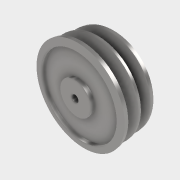
# Autodesk Inventor part: PWTR-0096
Saved by Autodesk Inventor 2021.1 (Build 251245000, 245)
## iProperties
CustomPartVersion: 1
Created: 2020-08-28
Part Number: PWTR-0096
Material: Stainless Steel
Document SubType Name: Modeling
Designer: alid
Density: 8 g/cm^3
Appearance: Semi-Polished
Description: Drive Unit Upper Pulley
Author: alid
Revision Number: A
Autodesk Inventor part; units mm, degrees
ref_plane "YZ Plane" through (0, 0, 0) normal (1, 0, 0) x (0, 1, 0)
ref_plane "XZ Plane" through (0, 0, 0) normal (0, 1, 0) x (-1, 0, 0)
sketch "Main Sketch" plane through (0, 0, 0) normal (1, 0, 0) x (0, 1, 0)
  line L0 (0, 28) -> (42, 28)
  line L1 (42, 28) -> (42, 12.8615)
  line L2 (42, 12.8615) -> (31, 9.4984)
  line L3 (31, 9.4984) -> (31, 6.5016)
  line L4 (31, 6.5016) -> (42, 3.1385)
  line L5 (42, 3.1385) -> (42, 0)
  line L6 (42, 0) -> (0, 0)
  line L7 (40, 12.25) -> (40, 3.75) construction
  line L8 (31, 8) -> (40, 8) construction
  line L9 (42, 12.8615) -> (42, 3.1385)
  line L10 (0, -5.6) -> (0, 33.6) projected
  line L11 (0, 0) -> (0, 28)
  line L12 (36, 0) -> (36, 3.5)
  line L13 (36, 3.5) -> (15, 3.5)
  line L14 (15, 3.5) -> (15, 0)
  line L15 (36, 28) -> (36, 24.5)
  line L16 (36, 24.5) -> (15, 24.5)
  line L17 (15, 24.5) -> (15, 28)
  dimension "d0" = 8.5
  dimension "d1" = 34
  dimension "d2" = 2
  dimension "d6" = 28
  dimension "d21" = 80
  dimension "d25" = 11
  dimension "d27" = 8
  dimension "d35" = 6
  dimension "d36" = 15
  dimension "d37" = 3.5
  constraints: 34 end point, 11 perpendicular, 6 point on line, 3 collinear, 2 equal length, 2 midpoint, 1 parallel
  measures "d0" distance of L7.start L7.end
  measures "d1" angle of L2 L4
  measures "d2" distance between parallel lines of L1 L7
  measures "d6" distance between parallel lines of L6 L0
  measures "d21" diameter of L7 L10
  measures "d25" distance between parallel lines of L3 L9
  measures "d27" distance between parallel lines of L6 L8
  measures "d35" distance between parallel lines of L5 L12
  measures "d36" distance between parallel lines of L10 L14
  measures "d37" distance of L13.end L14.end
ref_plane "Belt Plane" through (0, 31, 8) normal (0, 0, 1) x (1, 0, 0)
revolve "Body" add sketch "Main Sketch" angle 360 about axis through (0, 0, -10) along (0, 0, 1) contours L0 L17 L16 L15 L1 L2 L3 L4 L5 L6 L12 L13 L14 L10 | L9 L4 L3 L2
revolve "Groove" cut sketch "Main Sketch" angle 360 about axis through (0, 0, -10) along (0, 0, 1) contours L9 L4 L3 L2
fillet "Fillet External" [suppressed]
fillet "Fillet Internal" [suppressed]
pattern_linear "Groove Pattern" count 2 spacing 12 along (0, 0, 1) of "Groove"
sketch "Sketch2" plane through (0, 0, 0) normal (0, 0, -1) x (-1, 0, 0)
  circle A0 centre (0, 0) radius 42 projected
  constraints: 1 coincident
hole "Hole1" at (0, 0, 0) direction (0, 0, 1) diameter 6.6 end through all counterbore diameter 18 counterbore depth 23
equation "\"d0\" = da_Bw"
equation "\"d1\" = da_Alfa"
equation "\"d2\" = da_c"
equation "\"d21\" = da_Dw"
equation "\"d25\" = da_Hd"
equation "\"d27\" = da_Se"
equation "\"da_r1\" = 0"
equation "\"da_r2\" = 0"
equation "\"d18\" = da_Sg"
equation "\"d5\" = da_Se"
equation "\"da_Bw\" = 8.5"
equation "\"da_Alfa\" = 34deg"
equation "\"da_c\" = 2"
equation "\"da_Dw\" = 80"
equation "\"da_Hd\" = 11"
equation "\"da_Se\" = 8"
equation "\"da_Sg\" = 12"
body "Solid1"
